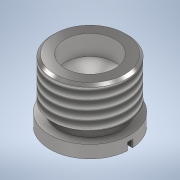
# Autodesk Inventor part: 2-螺塞
Saved by Autodesk Inventor 2022 (Build 260153000, 153)
## iProperties
Created: 2023-01-08
Part Number: 2-螺塞
Material: 不锈钢
Document SubType Name: Modeling
Designer: Lzy18
Density: 8 g/cm^3
Appearance: 半抛光
Author: Lzy18
Autodesk Inventor part; units mm, degrees
ref_plane "YZ Plane" through (0, 0, 0) normal (1, 0, 0) x (0, 1, 0)
ref_plane "XZ Plane" through (0, 0, 0) normal (0, 1, 0) x (-1, 0, 0)
ref_plane "XY Plane" through (0, 0, 0) normal (0, 0, 1) x (1, 0, 0)
sketch "草图1" plane through (0, 0, 0) normal (0, 1, 0) x (-1, 0, 0)
  circle A0 centre (0, 0) radius 16
  dimension "d0" = 32
  constraints: 1 centre point, 1 coincident
  measures "d0" diameter of A0
extrude "拉伸1" add sketch "草图1" along normal blind 5
sketch "草图2" plane through (0, 0, 0) normal (0, -1, 0) x (1, 0, 0)
  line L0 (16, 1) -> (-16, 1)
  line L1 (-16, 1) -> (-16, -1)
  line L2 (-16, -1) -> (16, -1)
  line L3 (16, -1) -> (16, 1)
  line L4 (16, 1) -> (-16, -1) construction
  line L5 (-16, 1) -> (16, -1) construction
  point P0 (0, 0)
  dimension "d3" = 32
  dimension "d4" = 2
  constraints: 12 end point, 2 midpoint, 2 parallel, 1 horizontal, 1 perpendicular
  measures "d3" distance of L2.end L1.end
  measures "d4" distance of L1.end L0.end
extrude "拉伸2" cut sketch "草图2" against normal blind 3
sketch "草图3" plane through (0, 5, 0) normal (0, 1, 0) x (1, 0, 0)
  circle A0 centre (0, 0) radius 12.5
  dimension "d7" = 25
  constraints: 1 centre point, 1 coincident
  measures "d7" diameter of A0
extrude "拉伸3" add sketch "草图3" along normal blind 4
sketch "草图4" plane through (0, 9, 0) normal (0, 1, 0) x (1, 0, 0)
  circle A0 centre (0, 0) radius 15
  dimension "d10" = 30
  constraints: 1 centre point, 1 coincident
  measures "d10" diameter of A0
extrude "拉伸4" add sketch "草图4" along normal blind 16
sketch "草图5" plane through (0, 25, 0) normal (0, 1, 0) x (1, 0, 0)
  circle A0 centre (0, 0) radius 10
  dimension "d13" = 20
  constraints: 1 centre point, 1 coincident
  measures "d13" diameter of A0
hole "孔1" at (0, 25, 0) direction (0, -1, 0) diameter 20 depth 8 tip angle 118
sketch "草图6" plane through (0, 0, 0) normal (1, 0, 0) x (0, 1, 0)
  line L0 (9, 15) -> (25, 15) projected
  line L1 (24, 15) -> (25, 14)
  line L2 (25, -15) -> (25, 15) projected
  line L3 (-5, 0) -> (30, 0) projected
  point P0 (0, 0)
  dimension "d21" = 1
  dimension "d22" = 45
  constraints: 2 end point, 2 point on line
  measures "d21" distance of L1.start L0.end
  measures "d22" angle of L0 L1
revolve "旋转1" cut sketch "草图6" angle 360 about axis through (0, -10, 0) along (0, 1, 0)
thread "螺纹1" size "M30x3.5" designation "M30" class "6g" standard "GB Metric profile" length 48
